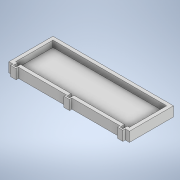
# Autodesk Inventor part: controllerBottom
Saved by Autodesk Inventor 2021 (Build 250183000, 183)
## iProperties
Created: 2024-03-19
Part Number: controllerBottom
Material: Generic
Document SubType Name: Modeling
Designer: 21seblin
Density: 1 g/cm^3
Appearance: Default
Author: 21seblin
Autodesk Inventor part; units mm, degrees
ref_plane "YZ Plane" through (0, 0, 0) normal (1, 0, 0) x (0, 1, 0)
ref_plane "XZ Plane" through (0, 0, 0) normal (0, 1, 0) x (-1, 0, 0)
ref_plane "XY Plane" through (0, 0, 0) normal (0, 0, 1) x (1, 0, 0)
sketch "Sketch1" plane through (0, 0, 0) normal (0, 1, 0) x (-1, 0, 0)
  line L0 (0, 0) -> (-175, 0)
  line L1 (-175, 0) -> (-175, 64)
  line L2 (-175, 64) -> (0, 64)
  line L3 (0, 64) -> (0, 0)
  line L4 (0, 64) -> (-6, 64)
  line L5 (-6, 64) -> (-14, 64)
  line L6 (-14, 64) -> (-14, 67.5)
  line L7 (-14, 67.5) -> (-6, 67.5)
  line L8 (-6, 67.5) -> (-6, 64)
  line L9 (-87.5, 64) -> (-87.5, 78.7696)
  line L10 (-87.5, 64) -> (-91.5, 64)
  line L11 (-91.5, 64) -> (-91.5, 65.75)
  line L12 (-83.5, 64) -> (-91.5, 64)
  line L13 (-83.5, 67.5) -> (-83.5, 64)
  line L14 (-91.5, 67.5) -> (-83.5, 67.5)
  line L15 (-91.5, 64) -> (-91.5, 67.5)
  line L16 (-161, 64) -> (-169, 64)
  line L17 (-161, 67.5) -> (-161, 64)
  line L18 (-169, 67.5) -> (-161, 67.5)
  line L19 (-169, 64) -> (-169, 67.5)
  dimension "d0" = 175
  dimension "d1" = 64
  dimension "d2" = 6
  dimension "d3" = 8
  dimension "d4" = 3.5
  dimension "d5" = 4
  dimension "d8" = 77.5
  constraints: 40 end point, 4 parallel, 3 horizontal, 2 perpendicular, 2 point on line, 2 vertical, 1 collinear, 1 midpoint, 15 other
  measures "d0" distance of L1.end L2.end
  measures "d1" distance of L0.end L1.end
  measures "d2" distance of L4.end L2.end
  measures "d3" distance of L6.end L7.end
  measures "d4" distance of L5.end L6.end
  measures "d5" distance of L10.end L9.start
  measures "d8" distance of L4.end L12.start
extrude "Extrusion1" add sketch "Sketch1" along normal blind 14
sketch "Sketch2" plane through (0, 14, 0) normal (0, 1, 0) x (1, 0, 0)
  line L0 (0, 0) -> (0, -64) projected
  line L1 (0, -6.5566) -> (5, -6.5566)
  line L2 (175, 0) -> (0, 0) projected
  line L3 (5, 0) -> (5, -5)
  line L4 (87.5, 0) -> (87.5, -64)
  line L5 (0, -32) -> (175, -32)
  line L6 (175, -64) -> (175, 0) projected
  line L7 (170, -59) -> (5, -59)
  line L8 (5, -59) -> (5, -5)
  line L9 (5, -5) -> (170, -5)
  line L10 (170, -5) -> (170, -59)
  line L11 (170, -59) -> (5, -5) construction
  line L12 (5, -59) -> (170, -5) construction
  line L13 (0, -64) -> (6, -64) projected
  line L14 (6, -64) -> (8, -64)
  line L15 (6, -67.5) -> (14, -67.5) projected
  line L16 (8, -67.5) -> (8, -65.5)
  line L17 (12, -62.5) -> (8, -62.5)
  line L18 (8, -62.5) -> (8, -65.5)
  line L19 (8, -65.5) -> (12, -65.5)
  line L20 (12, -65.5) -> (12, -62.5)
  line L21 (12, -62.5) -> (8, -65.5) construction
  line L22 (8, -62.5) -> (12, -65.5) construction
  line L23 (8, -59) -> (8, -62.5)
  line L24 (12, -59) -> (12, -62.5)
  line L25 (8, -59) -> (12, -59)
  line L26 (89.5, -59) -> (89.5, -62.5)
  line L27 (89.5, -65.5) -> (89.5, -62.5)
  line L28 (85.5, -65.5) -> (89.5, -65.5)
  line L29 (85.5, -62.5) -> (85.5, -65.5)
  line L30 (85.5, -59) -> (85.5, -62.5)
  line L31 (167, -59) -> (167, -62.5)
  line L32 (167, -65.5) -> (167, -62.5)
  line L33 (163, -65.5) -> (167, -65.5)
  line L34 (163, -62.5) -> (163, -65.5)
  line L35 (163, -59) -> (163, -62.5)
  point P0 (87.5, -32)
  point P1 (10, -64)
  dimension "d15" = 5
  dimension "d16" = 5
  dimension "d17" = 2
  dimension "d18" = 2
  dimension "d21" = 77.5
  constraints: 62 end point, 8 midpoint, 5 horizontal, 5 parallel, 5 point on line, 4 perpendicular, 2 collinear, 1 vertical, 21 other
  measures "d15" distance of L1.start L1.end
  measures "d16" distance of L3.start L3.end
  measures "d17" distance of L13.end L14.end
  measures "d18" distance of L16.start L16.end
  measures "d21" distance of L23.start L30.start
extrude "Extrusion2" cut sketch "Sketch2" against normal blind 9 contours L8 L9 L4 L5 | L5 L4 L7 L8 | L9 L10 L5 L4 | L5 L10 L7 L4 | L18 L17 L20 L19 | L7 L26 L27 L28 L29 L30 | L7 L24 L17 L23 | L7 L31 L32 L33 L34 L35
body "Solid1"
